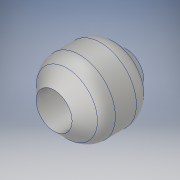
# Autodesk Inventor part: Handle
Saved by Autodesk Inventor 2019 Beta2 (Build 230110000, 110) ContinuousBuild 0
## iProperties
Created: 2015-04-24
Part Number: Handle
Material: Aluminum 6061
Document SubType Name: Modeling
Designer: John Helfen
Density: 2.7 g/cm^3
Appearance: Aluminum - Flat
Author: John Helfen
Autodesk Inventor part; units mm, degrees
ref_plane "YZ Plane" through (0, 0, 0) normal (1, 0, 0) x (0, 1, 0)
ref_plane "XZ Plane" through (0, 0, 0) normal (0, 1, 0) x (-1, 0, 0)
ref_plane "XY Plane" through (0, 0, 0) normal (0, 0, 1) x (1, 0, 0)
sketch "Sketch1" plane through (0, 0, 0) normal (0, 0, 1) x (1, 0, 0)
  circle A0 centre (0, 0) radius 3.175
  circle A1 centre (0, 0) radius 6.35
  dimension "d0" = 6.35
  dimension "d1" = 12.7
  constraints: 2 centre point, 2 coincident
  measures "d0" diameter of A0
  measures "d1" diameter of A1
extrude "Extrusion1" add sketch "Sketch1" against normal blind 12.7
chamfer "Chamfer1" distance 3.175 angle 45 2 edges at (-6.35, 0, 0) (-6.35, 0, -12.7)
fillet "Fillet1" radius 3.175 2 edges at (-6.35, 0, -3.1745) (-6.35, 0, -9.5255)
body "Solid1"
